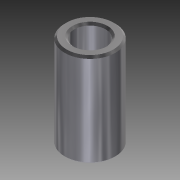
# Autodesk Inventor part: BearingLinearLMK8
Saved by Autodesk Inventor 2015 SP1 (Build 190203100, 203)
## iProperties
Category: Hardware
Created: 2014-10-10
Part Number: BearingLinearLMK8
Material: Steel, Alloy
Document SubType Name: Modeling
Designer: Jack
Density: 7.73 g/cm^3
Appearance: Semi-Polished
Mass: 15.1717 g
Surface Area: 17.0965 cm^2
Volume: 1.96271 cm^3
Vendor: Misumi
Author: Jack
Title: Bearing LMK8
Autodesk Inventor part; units mm, degrees
ref_plane "YZ Plane" through (0, 0, 0) normal (1, 0, 0) x (0, 1, 0)
ref_plane "XZ Plane" through (0, 0, 0) normal (0, 1, 0) x (-1, 0, 0)
ref_plane "XY Plane" through (0, 0, 0) normal (0, 0, 1) x (1, 0, 0)
sketch "Sketch1" plane through (0, 0, 0) normal (0, 0, 1) x (1, 0, 0)
  circle A0 centre (0, 0) radius 4
  circle A1 centre (0, 0) radius 6.5
  dimension "d0" = 8
  dimension "d1" = 13
  constraints: 2 centre point, 2 coincident
  measures "d0" diameter of A0
  measures "d1" diameter of A1
extrude "Extrusion1" add sketch "Sketch1" along normal blind 24
chamfer "Chamfer1" distance 0.5 angle 45 4 edges at (-6.5, 0, 24) (-4, 0, 24) (-6.5, 0, 0) (-4, 0, 0)
body "Solid1"
